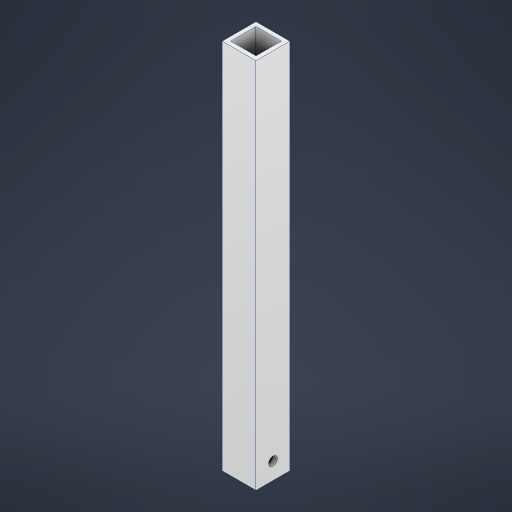
# Autodesk Inventor part: STRU_010_BilletPole_11in_Unique
Saved by Autodesk Inventor 2024.2 (Build 282272000, 272)
## iProperties
Created: 2024-07-23
Part Number: STRU_010_BilletPole_11in_Unique
Material: Aluminum 6061
Document SubType Name: Modeling
Designer: bryan
Density: 2.7 g/cm^3
Appearance: Aluminum - Flat
Mass: 212.929 g
Surface Area: 502.418 cm^2
Volume: 78.8627 cm^3
Author: bryan
Autodesk Inventor part; units mm, degrees
ref_plane "YZ Plane" through (0, 0, 0) normal (1, 0, 0) x (0, 1, 0)
ref_plane "XZ Plane" through (0, 0, 0) normal (0, 1, 0) x (-1, 0, 0)
ref_plane "XY Plane" through (0, 0, 0) normal (0, 0, 1) x (1, 0, 0)
sketch "Sketch1" plane through (0, 0, 0) normal (0, 1, 0) x (-1, 0, 0)
  line L0 (-12.7, -12.7) -> (12.7, -12.7)
  line L1 (12.7, -12.7) -> (12.7, 12.7)
  line L2 (12.7, 12.7) -> (-12.7, 12.7)
  line L3 (-12.7, 12.7) -> (-12.7, -12.7)
  line L4 (-12.7, -12.7) -> (12.7, 12.7) construction
  line L5 (12.7, -12.7) -> (-12.7, 12.7) construction
  line L6 (9.525, 9.525) -> (9.525, -9.525)
  line L7 (9.525, -9.525) -> (-9.525, -9.525)
  line L8 (-9.525, -9.525) -> (-9.525, 9.525)
  line L9 (-9.525, 9.525) -> (9.525, 9.525)
  point P0 (0, 0)
  dimension "d0" = 25.4
  dimension "d1" = 25.4
  dimension "d2" = 3.175
  constraints: 20 end point, 4 parallel, 2 midpoint, 2 perpendicular, 1 horizontal, 3 other
  measures "d0" distance of L2.end L1.end
  measures "d1" distance of L1.end L0.end
  measures "d2" distance between parallel lines of L1 L6
extrude "Extrusion1" add sketch "Sketch1" along normal blind 279.4
sketch "Sketch2" plane through (12.7, 0, 12.7) normal (1, 0, 0) x (0, 0, -1)
  circle A0 centre (12.7, 12.7) radius 3.2512
  line L0 (0, 0) -> (25.4, 0) projected
  point P0 (12.7, 0)
  point P1 (12.7, 0)
  point P2 (12.7, 0)
  dimension "d5" = 6.5024
  dimension "d6" = 12.7
  constraints: 2 midpoint, 1 centre point, 1 vertical alignment
  measures "d5" diameter of A0
  measures "d6" distance of point (12.7, 0) A0.centre
extrude "Extrusion2" cut sketch "Sketch2" against normal blind 25.4
body "Solid1"
